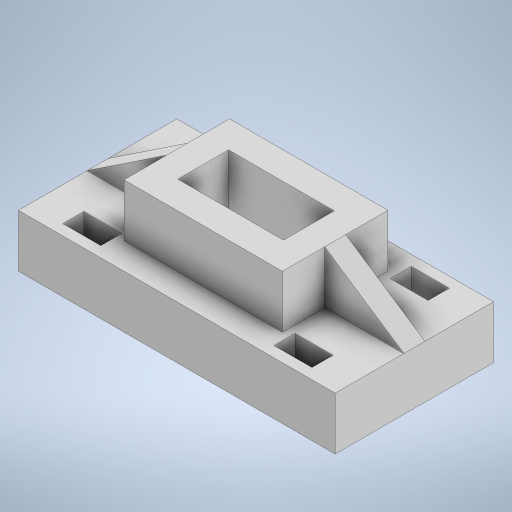
# Autodesk Inventor part: 6 - Part 3
Saved by Autodesk Inventor 2024 (Build 280153000, 153)
## iProperties
Created: 2024-04-21
Part Number: 6 - Part 3
Material: Generic
Document SubType Name: Modeling
Designer: Ricsi
Density: 1 g/cm^3
Appearance: Default
Author: Ricsi
Autodesk Inventor part; units mm, degrees
ref_plane "YZ Plane" through (0, 0, 0) normal (1, 0, 0) x (0, 1, 0)
ref_plane "XZ Plane" through (0, 0, 0) normal (0, 1, 0) x (-1, 0, 0)
ref_plane "XY Plane" through (0, 0, 0) normal (0, 0, 1) x (1, 0, 0)
sketch "Sketch1" plane through (0, 0, 0) normal (0, 1, 0) x (-1, 0, 0)
  line L0 (0, 93.9079) -> (150, 93.9079)
  line L1 (150, 93.9079) -> (150, 168.9079)
  line L2 (150, 168.9079) -> (0, 168.9079)
  line L3 (0, 168.9079) -> (0, 93.9079)
  point P0 (0, 0)
  dimension "d0" = 150
  dimension "d1" = 75
  constraints: 8 end point, 2 parallel, 1 horizontal, 1 perpendicular
  measures "d0" distance of L2.end L1.end
  measures "d1" distance of L1.end L0.end
extrude "Extrusion1" add sketch "Sketch1" along normal blind 25
sketch "Sketch2" plane through (0, 25, 0) normal (0, 1, 0) x (1, 0, 0)
  line L0 (0, -168.9079) -> (-75, -168.9079)
  line L1 (-75, -156.4079) -> (-112.5, -156.4079)
  line L2 (-75, -156.4079) -> (-37.5, -156.4079)
  line L3 (-37.5, -156.4079) -> (-37.5, -106.4079)
  line L4 (-37.5, -106.4079) -> (-112.5, -106.4079)
  line L5 (-112.5, -106.4079) -> (-112.5, -156.4079)
  point P0 (0, 0)
  dimension "d8" = 37.5
  dimension "d9" = 37.5
  dimension "d10" = 50
  dimension "d11" = 75
  constraints: 12 end point, 3 horizontal, 1 vertical
  measures "d8" distance of L1.start L1.end
  measures "d9" distance of L1.start L2.end
  measures "d10" distance of L2.end L3.end
  measures "d11" distance of L3.end L4.end
extrude "Extrusion2" add sketch "Sketch2" along normal blind 25
sketch "Sketch3" plane through (0, 50, 0) normal (0, 1, 0) x (1, 0, 0)
  line L0 (-112.5, -156.4079) -> (-37.5, -156.4079) projected
  line L1 (-37.5, -156.4079) -> (-37.5, -131.4079)
  line L2 (-75, -143.4079) -> (-100, -143.4079)
  line L3 (-75, -143.4079) -> (-50, -143.4079)
  line L4 (-50, -143.4079) -> (-50, -119.4079)
  line L5 (-50, -119.4079) -> (-100, -119.4079)
  line L6 (-100, -143.4079) -> (-100, -119.4079)
  point P0 (0, 0)
  dimension "d18" = 25
  dimension "d19" = 25
  dimension "d20" = 24
  dimension "d21" = 50
  constraints: 12 end point, 3 horizontal, 2 vertical
  measures "d18" distance of L2.start L2.end
  measures "d19" distance of L2.start L3.end
  measures "d20" distance of L3.end L4.end
  measures "d21" distance of L4.end L5.end
extrude "Extrusion3" cut sketch "Sketch3" against normal blind 30
sketch "Sketch4" plane through (0, 25, 0) normal (0, 1, 0) x (1, 0, 0)
  line L0 (-37.5, -106.4079) -> (-37.5, -156.4079) projected
  line L1 (-37.5, -156.4079) -> (-37.5, -131.4079)
  line L2 (-37.5, -131.4079) -> (-37.5, -126.4079)
  line L3 (-37.5, -131.4079) -> (-37.5, -136.4079)
  line L4 (-37.5, -136.4079) -> (0, -136.4079)
  line L5 (0, -168.9079) -> (0, -93.9079) projected
  line L6 (0, -136.4079) -> (0, -126.4079)
  line L7 (0, -126.4079) -> (-37.5, -126.4079)
  line L8 (-112.5, -156.4079) -> (-112.5, -106.4079) projected
  line L9 (-112.5, -106.4079) -> (-112.5, -131.4079)
  line L10 (-37.5, -156.4079) -> (-112.5, -156.4079) projected
  line L11 (-112.5, -131.4079) -> (-112.5, -136.4079)
  line L12 (-112.5, -131.4079) -> (-112.5, -126.4079)
  line L13 (-112.5, -136.4079) -> (-150, -136.4079)
  line L14 (-150, -93.9079) -> (-150, -168.9079) projected
  line L15 (-150, -136.4079) -> (-150, -126.4079)
  line L16 (-150, -126.4079) -> (-112.5, -126.4079)
  point P0 (0, 0)
  dimension "d25" = 5
  dimension "d26" = 5
  dimension "d27" = 10
  dimension "d29" = 5
  dimension "d30" = 5
  dimension "d31" = 10
  constraints: 24 end point, 7 point on line, 2 horizontal, 2 perpendicular, 1 midpoint
  measures "d25" distance of L1.end L2.end
  measures "d26" distance of L1.end L3.end
  measures "d27" distance of L4.end L6.end
  measures "d29" distance of L9.end L11.end
  measures "d30" distance of L9.end L12.end
  measures "d31" distance of L13.end L15.end
extrude "Extrusion4" add sketch "Sketch4" along normal blind 25
sketch "Sketch5" plane through (-150, 25, 136.4079) normal (0, 0, 1) x (1, 0, 0)
  line L0 (37.5, 25) -> (0, 0)
  line L1 (0, 25) -> (37.5, 25) projected
  line L2 (0, 0) -> (0, 25)
  line L3 (0, 25) -> (37.5, 25)
  point P0 (150, -25)
  constraints: 6 end point, 1 collinear, 1 perpendicular
extrude "Extrusion5" cut sketch "Sketch5" against normal blind 25
sketch "Sketch6" plane through (-37.5, 25, 136.4079) normal (0, 0, 1) x (1, 0, 0)
  line L0 (0, 25) -> (37.5, 25) projected
  line L1 (37.5, 0) -> (0, 0) projected
  line L2 (0, 25) -> (37.5, 0)
  line L3 (37.5, 0) -> (37.5, 25) projected
  line L4 (37.5, 0) -> (37.5, 25)
  line L5 (37.5, 25) -> (0, 25)
  point P0 (37.5, -25)
  constraints: 6 end point, 1 collinear, 1 perpendicular, 1 point on line
extrude "Extrusion6" cut sketch "Sketch6" against normal blind 25
sketch "Sketch7" plane through (0, 25, 0) normal (0, 1, 0) x (1, 0, 0)
  line L0 (0, -126.4079) -> (0, -93.9079) projected
  line L1 (0, -93.9079) -> (-25, -93.9079)
  line L2 (-34, -103.9079) -> (-34, -98.9079)
  line L3 (-34, -103.9079) -> (-34, -108.9079)
  line L4 (-34, -108.9079) -> (-16, -108.9079)
  line L5 (-16, -108.9079) -> (-16, -98.9079)
  line L6 (-16, -98.9079) -> (-34, -98.9079)
  line L7 (-150, -93.9079) -> (-116, -93.9079)
  line L8 (-116, -98.9079) -> (-116, -108.9079)
  line L9 (-116, -108.9079) -> (-134, -108.9079)
  line L10 (-134, -108.9079) -> (-134, -98.9079)
  line L11 (-134, -98.9079) -> (-116, -98.9079)
  line L12 (-116, -153.9079) -> (-116, -163.9079)
  line L13 (-116, -163.9079) -> (-134, -163.9079)
  line L14 (-134, -163.9079) -> (-134, -153.9079)
  line L15 (-134, -153.9079) -> (-116, -153.9079)
  line L16 (-150, -168.9079) -> (0, -168.9079) projected
  line L17 (-150, -136.4079) -> (-150, -168.9079) projected
  line L18 (-16, -153.9079) -> (-16, -163.9079)
  line L19 (-16, -163.9079) -> (-34, -163.9079)
  line L20 (-34, -163.9079) -> (-34, -153.9079)
  line L21 (-34, -153.9079) -> (-16, -153.9079)
  line L22 (0, -168.9079) -> (0, -136.4079) projected
  point P0 (0, 0)
  dimension "d44" = 5
  dimension "d45" = 5
  dimension "d46" = 18
  dimension "d47" = 10
  dimension "d50" = 10
  dimension "d51" = 18
  dimension "d52" = 10
  dimension "d53" = 10
  dimension "d54" = 18
  dimension "d55" = 10
  dimension "d56" = 5
  dimension "d57" = 16
  dimension "d58" = 10
  dimension "d59" = 18
  dimension "d60" = 10
  dimension "d61" = 16
  dimension "d62" = 5
  constraints: 38 end point, 9 vertical, 4 horizontal
  measures "d44" distance of L2.start L2.end
  measures "d45" distance of L2.start L3.end
  measures "d46" distance of L3.end L4.end
  measures "d47" distance of L4.end L5.end
  measures "d50" distance of L8.start L8.end
  measures "d51" distance of L8.end L9.end
  measures "d52" distance of L9.end L10.end
  measures "d53" distance of L12.start L12.end
  measures "d54" distance of L12.end L13.end
  measures "d55" distance of L13.end L14.end
  measures "d56" distance between parallel lines of L13 L16
  measures "d57" distance between parallel lines of L17 L14
  measures "d58" distance of L21.end L19.start
  measures "d59" distance of L19.start L19.end
  measures "d60" distance of L19.end L21.start
  measures "d61" distance between parallel lines of L22 L18
  measures "d62" distance between parallel lines of L19 L16
extrude "Extrusion7" cut sketch "Sketch7" against normal blind 25
body "Solid1"
